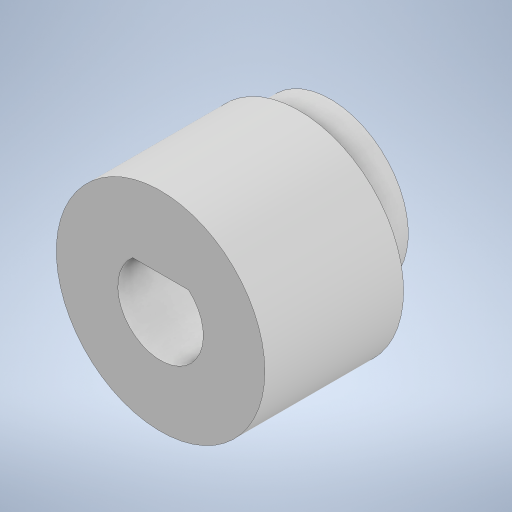
# Autodesk Inventor part: 감속기어1 - 축
Saved by Autodesk Inventor 2023 (Build 270158000, 158)
## iProperties
Created: 2022-06-21
Part Number: 감속기어1 - 축
Material: 일반
Document SubType Name: Modeling
Designer: user
Density: 1 g/cm^3
Appearance: 기본값
Author: user
Autodesk Inventor part; units mm, degrees
ref_plane "YZ Plane" through (0, 0, 0) normal (1, 0, 0) x (0, 1, 0)
ref_plane "XZ Plane" through (0, 0, 0) normal (0, 1, 0) x (-1, 0, 0)
ref_plane "XY Plane" through (0, 0, 0) normal (0, 0, 1) x (1, 0, 0)
sketch "스케치1" plane through (0, 0, 0) normal (0, 0, 1) x (1, 0, 0)
  circle A0 centre (0, 0) radius 10
  circle A1 centre (0, 0) radius 4
  dimension "d0" = 20
  dimension "d1" = 8
  constraints: 2 centre point, 2 coincident
  measures "d0" diameter of A0
  measures "d1" diameter of A1
extrude "돌출1" add sketch "스케치1" along normal blind 13.3
sketch "스케치2" plane through (0, 0, 0) normal (0, 0, -1) x (-1, 0, 0)
  line L0 (-2.6458, 3) -> (2.6458, 3)
  circle A0 centre (0, 0) radius 4 projected
  dimension "d4" = 3
  constraints: 2 end point, 2 point on circle, 1 horizontal
  measures "d4" distance from line of point (0, 0) L0
extrude "돌출2" add sketch "스케치2" against normal up to surface (13.3 mm away) contours A0 L0 picked at (-0.6179, 3.1815)
sketch "스케치3" plane through (0, 0, 0) normal (0, 0, -1) x (-1, 0, 0)
  circle A0 centre (2, 0) radius 7.45
  line L0 (0, 0) -> (2, 0)
  arc A1 (-2.6458, 3) -> (2.6458, 3) centre (0, 0) ccw projected
  line L1 (-2.6458, 3) -> (2.6458, 3) projected
  dimension "d7" = 14.9
  dimension "d8" = 2
  constraints: 2 end point, 1 centre point, 1 horizontal
  measures "d7" diameter of A0
  measures "d8" distance of L0.start L0.end
extrude "돌출3" add sketch "스케치3" along normal blind 5
sketch "스케치4" plane through (-2, 0, -5) normal (0, 0, -1) x (-1, 0, 0)
  arc A0 (-4.6458, 3) -> (0.6458, 3) centre (-2, 0) ccw projected
  line L0 (-4.6458, 3) -> (0.6458, 3) projected
  arc A1 (-4.6833, 3.1) -> (0.6833, 3.1) centre (-2, 0) ccw
  line L1 (-4.6833, 3.1) -> (0.6833, 3.1)
  dimension "d11" = 0.1
  constraints: 2 end point, 2 point on circle, 1 centre point, 1 other
  measures "d11" radial gap between concentric circles of A0 A1
extrude "돌출4" cut sketch "스케치4" against normal up to surface (18.3 mm away) contours L0 A0 | L1 A1
